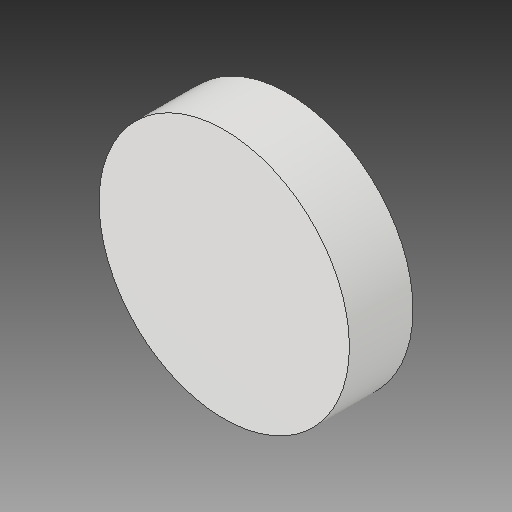
# Autodesk Inventor part: Button
Saved by Autodesk Inventor 2019 (Build 230136000, 136)
## iProperties
Created: 2018-09-21
Part Number: Button
Material: ABS Plastic
Document SubType Name: Modeling
Designer: user
Density: 1.06 g/cm^3
Appearance: Smooth - White
Author: user
Autodesk Inventor part; units mm, degrees
ref_plane "YZ Plane" through (0, 0, 0) normal (1, 0, 0) x (0, 1, 0)
ref_plane "XZ Plane" through (0, 0, 0) normal (0, 1, 0) x (-1, 0, 0)
ref_plane "XY Plane" through (0, 0, 0) normal (0, 0, 1) x (1, 0, 0)
sketch "Sketch1" plane through (0, 0, 0) normal (0, 0, 1) x (1, 0, 0)
  circle A0 centre (165.1, 914.4) radius 30
  line L0 (228.6, 1219.2) -> (-228.6, 1219.2) projected
  line L1 (-228.6, 1219.2) -> (-228.6, -1219.2) projected
  line L2 (-228.6, -1219.2) -> (228.6, -1219.2) projected
  line L3 (228.6, -1219.2) -> (228.6, 1219.2) projected
  line L4 (101.6, 889) -> (101.6, 1219.2) projected
  point P0 (0, 0)
  dimension "d0" = 63.5
  dimension "d1" = 304.8
  dimension "d2" = 60
  constraints: 1 centre point
  measures "d0" distance from line of L4 A0.centre
  measures "d1" distance from line of L0 A0.centre
  measures "d2" diameter of A0
extrude "Extrusion1" add sketch "Sketch1" along normal blind 15.24 contours A0
body "Solid1"
